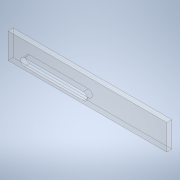
# Autodesk Inventor part: Electronics Side Plate Holes
Saved by Autodesk Inventor 2022 (Build 260153000, 153)
## iProperties
Created: 2022-01-15
Part Number: Electronics Side Plate Holes
Material: Generic
Document SubType Name: Modeling
Designer: merky
Density: 1 g/cm^3
Appearance: Polycarbonate - Clear
Author: merky
Autodesk Inventor part; units mm, degrees
ref_plane "YZ Plane" through (0, 0, 0) normal (1, 0, 0) x (0, 1, 0)
ref_plane "XZ Plane" through (0, 0, 0) normal (0, 1, 0) x (-1, 0, 0)
ref_plane "XY Plane" through (0, 0, 0) normal (0, 0, 1) x (1, 0, 0)
sketch "Sketch1" plane through (0, 0, 0) normal (0, 0, 1) x (1, 0, 0)
  line L0 (0, 0) -> (393.7, 0)
  line L1 (393.7, 0) -> (393.7, 63.5)
  line L2 (393.7, 63.5) -> (0, 63.5)
  line L3 (0, 63.5) -> (0, 0)
  dimension "d0" = 393.7
  dimension "d1" = 63.5
  constraints: 8 end point, 2 parallel, 1 horizontal, 1 perpendicular
  measures "d0" distance of L2.end L1.end
  measures "d1" distance of L1.end L0.end
extrude "Extrusion1" add sketch "Sketch1" along normal blind 12.7
sketch "Sketch2" plane through (0, 0, 12.7) normal (0, 0, 1) x (1, 0, 0)
  line L0 (40.7802, 26.1158) -> (186.8302, 26.1158)
  line L1 (196.3552, 16.5908) -> (196.3552, 16.5908)
  line L2 (186.8302, 7.0658) -> (40.7802, 7.0658)
  line L3 (31.2552, 16.5908) -> (31.2552, 16.5908)
  arc A0 (40.7802, 26.1158) -> (31.2552, 16.5908) centre (40.7802, 16.5908) ccw
  arc A1 (31.2552, 16.5908) -> (40.7802, 7.0658) centre (40.7802, 16.5908) ccw
  arc A2 (186.8302, 7.0658) -> (196.3552, 16.5908) centre (186.8302, 16.5908) ccw
  arc A3 (196.3552, 16.5908) -> (186.8302, 26.1158) centre (186.8302, 16.5908) ccw
  point P0 (196.3552, 7.0658)
  point P1 (196.3552, 26.1158)
  point P2 (31.2552, 7.0658)
  point P3 (31.2552, 16.5908)
  dimension "d4" = 165.1
  dimension "d5" = 19.05
  dimension "d6" = 9.525
  constraints: 8 end point, 8 point on circle, 8 tangent, 6 point on line, 4 centre point, 3 equal radius, 2 parallel, 1 horizontal, 1 perpendicular
  measures "d4" distance of point (196.355, 7.066) point (31.255, 7.066)
  measures "d5" distance of point (196.355, 26.116) point (196.355, 7.066)
  measures "d6" radius of A0
extrude "Extrusion2" cut sketch "Sketch2" against normal through all
body "Solid1"
